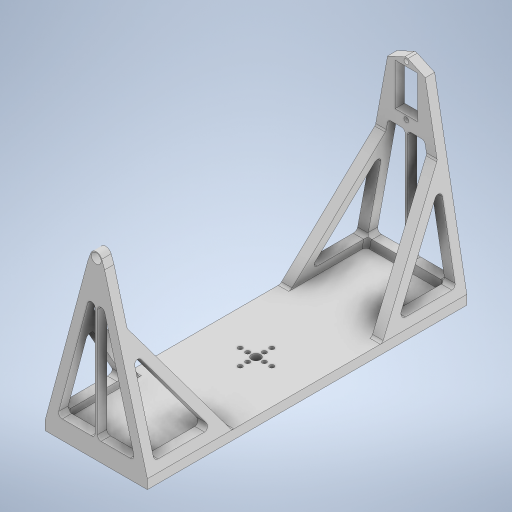
# Autodesk Inventor part: holder
Saved by Autodesk Inventor 2024 (Build 280153000, 153)
## iProperties
Created: 2025-03-10
Part Number: holder
Material: Generic
Document SubType Name: Modeling
Designer: 5454s
Density: 1 g/cm^3
Appearance: Default
Author: 5454s
Autodesk Inventor part; units mm, degrees
ref_plane "YZ Plane" through (0, 0, 0) normal (1, 0, 0) x (0, 1, 0)
ref_plane "XZ Plane" through (0, 0, 0) normal (0, 1, 0) x (-1, 0, 0)
ref_plane "XY Plane" through (0, 0, 0) normal (0, 0, 1) x (1, 0, 0)
sketch "Sketch1" plane through (0, 0, 0) normal (0, 0, 1) x (1, 0, 0)
  line L0 (0, 0) -> (8.8545, 0)
  line L1 (8.8545, 0) -> (8.8545, 85)
  line L2 (8.8545, 85) -> (0, 85)
  line L3 (0, 85) -> (0, 0)
  line L4 (0, 85) -> (-22.7757, 0)
  line L5 (-22.7757, 0) -> (31.6302, 0)
  line L6 (31.6302, 0) -> (8.8545, 85)
  circle A0 centre (4.4273, 88.1) radius 3.1
  line L7 (4.4273, 0) -> (4.4273, 91.736)
  line L8 (7.5273, 88.1) -> (1.3273, 88.1)
  circle A1 centre (4.4273, 88.1) radius 2.6
  line L9 (4.4273, 88.1) -> (1.5142, 89.1603)
  line L10 (1.5142, 89.1603) -> (0, 85)
  line L11 (4.4273, 88.1) -> (7.3403, 89.1603)
  line L12 (7.3403, 89.1603) -> (8.8545, 85)
  line L13 (-16.2596, 5) -> (4.4273, 5)
  line L14 (3.8366, 80) -> (-16.2596, 5)
  line L15 (3.8366, 80) -> (4.4273, 80)
  line L16 (4.4273, 80) -> (5.0179, 80)
  line L17 (5.0179, 80) -> (25.1141, 5)
  line L18 (25.1141, 5) -> (4.4273, 5)
  line L19 (3.8366, 80) -> (3.8366, 5)
  line L20 (5.0179, 80) -> (5.0179, 5)
  point P0 (0, 42.5)
  point P1 (-15.2073, 5)
  point P2 (20.2424, 42.5)
  dimension "d0" = 85
  dimension "d1" = 75
  dimension "d2" = 75
  dimension "d4" = 6.2
  dimension "d6" = 5.2
  dimension "d7" = 20
  dimension "d8" = 70
  dimension "d9" = 20
  dimension "d10" = 70
  dimension "d15" = 54.4059
  dimension "d22" = 5
  dimension "d27" = 5
  dimension "d28" = 5
  constraints: 42 end point, 6 horizontal, 6 point on line, 4 midpoint, 4 perpendicular, 4 point on circle, 2 centre point, 2 parallel, 1 coincident, 1 collinear, 1 tangent, 1 vertical, 1 other
  measures "d0" distance of L0.end L1.end
  measures "d1" angle of L5 L6
  measures "d2" angle of L5 L4
  measures "d4" diameter of A0
  measures "d6" diameter of A1
  measures "d7" angle of L8 L9
  measures "d8" angle of L2 L10
  measures "d9" angle of L8 L11
  measures "d10" angle of L2 L12
  measures "d15" distance of L5.end L4.end
  measures "d22" distance between parallel lines of L5 L13
  measures "d27" distance between parallel lines of L4 L14
  measures "d28" distance between parallel lines of L2 L15
extrude "Extrusion1" add sketch "Sketch1" along normal blind 5 contours L3 L13 L7 L0 | L5 L4 L3 L14 L13 | L7 L18 L1 L0 | L1 L18 L17 L6 L5 | L13 L19 L15 L7 | L7 L16 L20 L18 | L3 L2 L7 L15 L14 | L10 A0 L2 | L7 L2 L1 L17 L16 | A0 L12 L2 | L7 A1 L8 A0 | A0 L8 A1 L7 | L9 A1 L8 A0 | A0 L7 A1 L9 | L8 A1 L11 A0 | A0 L11 A1 L7
fillet "Fillet1" radius 2 6 edges at (5.0179, 5, 2.5) (-16.2596, 5, 2.5) (3.8366, 5, 2.5) (25.1141, 5, 2.5) (3.8366, 80, 2.5) (5.0179, 80, 2.5)
sketch "Sketch2" plane through (-22.7757, 0, 0) normal (0, -1, 0) x (1, 0, 0)
  line L0 (0, 0) -> (54.4059, 0) projected
  line L1 (54.4059, 0) -> (54.4059, 5) projected
  line L2 (0, 5) -> (54.4059, 5) projected
  line L3 (0, 0) -> (0, 5) projected
  line L4 (0, 0) -> (54.4059, 0)
  line L5 (54.4059, 0) -> (54.4059, -144.177)
  line L6 (54.4059, -144.177) -> (0, -144.177)
  line L7 (0, -144.177) -> (0, 0)
  line L8 (54.4059, 0) -> (54.4059, 5) projected
  line L9 (54.4059, -144.177) -> (0, -144.177)
  line L10 (0, -144.177) -> (0, -165.177)
  line L11 (0, -165.177) -> (54.4059, -165.177)
  line L12 (54.4059, -165.177) -> (54.4059, -144.177)
  point P0 (22.7757, 0)
  dimension "d32" = 144.177
  dimension "d34" = 21
  constraints: 16 end point, 4 parallel, 2 collinear, 2 horizontal, 2 perpendicular
  measures "d32" distance of L4.end L5.end
  measures "d34" distance of L9.end L10.end
extrude "Extrusion2" add sketch "Sketch2" along normal blind 5
sketch "Sketch5" plane through (-22.7757, 0, 0) normal (0, 1, 0) x (1, 0, 0)
  line L0 (0, 0) -> (54.4059, 0) projected
  line L1 (54.4059, 165.177) -> (54.4059, 0) projected
  line L2 (0, 165.177) -> (54.4059, 165.177) projected
  line L3 (0, 0) -> (0, 165.177) projected
  line L4 (54.4059, 165.177) -> (0, 165.177)
  line L5 (0, 165.177) -> (0, 160.177)
  line L6 (0, 160.177) -> (54.4059, 160.177)
  line L7 (54.4059, 160.177) -> (54.4059, 165.177)
  point P0 (22.7757, 0)
  dimension "d37" = 5
  constraints: 8 end point, 2 parallel, 1 horizontal, 1 perpendicular, 1 point on line
  measures "d37" distance between parallel lines of L2 L6
extrude "Extrusion3" add sketch "Sketch5" along normal up to surface (91.2 mm away) contours L3 L2 L1 L6
sketch "Sketch9" plane through (31.6302, -5, -165.177) normal (0, 0, -1) x (-1, 0, 0)
  line L0 (31.6302, 90) -> (54.4059, 5) projected
  line L1 (0, 5) -> (22.7757, 90) projected
  circle A0 centre (27.2029, 93.1) radius 2.6 projected
  line L2 (30.116, 94.1603) -> (31.6302, 90) projected
  line L3 (22.7757, 90) -> (24.2899, 94.1603) projected
  arc A1 (30.116, 94.1603) -> (24.2899, 94.1603) centre (27.2029, 93.1) ccw projected
  circle A2 centre (27.2029, 101.3) radius 1.25
  circle A3 centre (27.2029, 74.5) radius 1.25
  line L4 (21.2029, 76.6) -> (33.2029, 76.6)
  line L5 (33.2029, 76.6) -> (33.2029, 99)
  line L6 (33.2029, 99) -> (21.2029, 99)
  line L7 (21.2029, 99) -> (21.2029, 76.6)
  line L8 (0, 5) -> (17.1194, 98.9034)
  circle A4 centre (27.2029, 101.3) radius 2
  line L9 (0, 5) -> (54.4059, 5) projected
  line L10 (25.2029, 101.3) -> (29.2029, 101.3)
  line L11 (27.2029, 101.3) -> (26.3577, 103.1126)
  line L12 (26.3577, 103.1126) -> (17.1194, 98.9034)
  line L13 (27.2029, 101.3) -> (28.0482, 103.1126)
  line L14 (54.4059, 5) -> (37.2029, 98.8882)
  line L15 (28.0482, 103.1126) -> (37.2029, 98.8882)
  point P0 (31.6302, 5)
  point P1 (27.2029, 99)
  point P2 (21.2029, 84.1305)
  point P3 (33.2029, 84.1305)
  dimension "d54" = 8.2
  dimension "d55" = 18.6
  dimension "d56" = 12
  dimension "d57" = 22.4
  dimension "d58" = 2.5
  dimension "d59" = 2.3
  dimension "d60" = 4
  dimension "d62" = 4
  dimension "d63" = 79.668
  dimension "d64" = 65
  dimension "d65" = 65
  dimension "d66" = 124.827
  dimension "d67" = 4
  constraints: 22 end point, 4 point on circle, 3 centre point, 3 vertical alignment, 2 horizontal, 2 parallel, 1 coincident, 1 equal length, 1 equal radius, 1 midpoint, 1 perpendicular
  measures "d54" distance of A0.centre A2.centre
  measures "d55" distance of A3.centre A0.centre
  measures "d56" distance of L4.start L4.end
  measures "d57" distance of L4.end L5.end
  measures "d58" diameter of A2
  measures "d59" distance from line of A2.centre L6
  measures "d60" distance from line of L8 L6.end
  measures "d62" diameter of A4
  measures "d63" angle of L9 L8
  measures "d64" angle of L10 L11
  measures "d65" angle of L10 L13
  measures "d66" angle of L8 L12
  measures "d67" horizontal distance of L14.end L5.end
extrude "Extrusion6" add sketch "Sketch9" against normal up to surface (5 mm away) contours L5 L6 L7 L1 L8 L12 A4 L15 L14 L0 | L13 A2 L11 A4 | A4 L10 A2 L13 | L11 A2 L10 A4 | A4 L10 A2
sketch "Sketch10" plane through (31.6302, -5, -165.177) normal (0, 0, -1) x (-1, 0, 0)
  line L0 (16.6265, 96.2) -> (0, 96.2) projected
  line L1 (0, 96.2) -> (0, 0) projected
  line L2 (54.4059, 0) -> (0, 0) projected
  line L3 (54.4059, 96.2) -> (54.4059, 0) projected
  line L4 (54.4059, 96.2) -> (37.6955, 96.2) projected
  line L5 (37.6955, 96.2) -> (37.2029, 98.8882) projected
  line L6 (37.2029, 98.8882) -> (28.0482, 103.1126) projected
  arc A0 (28.0482, 103.1126) -> (26.3577, 103.1126) centre (27.2029, 101.3) ccw projected
  line L7 (26.3577, 103.1126) -> (17.1194, 98.9034) projected
  line L8 (17.1194, 98.9034) -> (16.6265, 96.2) projected
  circle A1 centre (27.2029, 101.3) radius 1.25 projected
  line L9 (21.2029, 96.2) -> (21.2029, 99) projected
  line L10 (21.2029, 99) -> (33.2029, 99) projected
  line L11 (33.2029, 99) -> (33.2029, 96.2) projected
  line L12 (33.2029, 96.2) -> (21.2029, 96.2) projected
  line L13 (21.2029, 99) -> (33.2029, 99)
  line L14 (33.2029, 99) -> (33.2029, 76.6)
  line L15 (33.2029, 76.6) -> (21.2029, 76.6)
  line L16 (21.2029, 76.6) -> (21.2029, 99)
  circle A2 centre (27.2029, 74.5) radius 1.25
  circle A3 centre (27.2029, 101.3) radius 1.25 projected
  line L17 (31.6302, 90) -> (54.4059, 5) projected
  line L18 (0, 5) -> (22.7757, 90) projected
  line L19 (0, 5) -> (54.4059, 5) projected
  line L20 (17.1194, 98.9034) -> (0, 5)
  line L21 (37.2029, 98.8882) -> (54.4059, 5)
  point P0 (31.6302, 5)
  point P1 (37.6955, 96.2)
  point P2 (21.2029, 96.2)
  dimension "d70" = 22.4
  dimension "d71" = 26.8
  constraints: 12 end point, 2 parallel, 1 centre point, 1 equal radius, 1 horizontal, 1 perpendicular, 1 vertical alignment
  measures "d70" distance of L10.end L14.end
  measures "d71" distance of A2.centre A0.centre
extrude "Extrusion7" cut sketch "Sketch10" against normal blind 10 contours L20 L1 L0 | L16 L12 L14 L15 | L21 L4 L3 | A2
sketch "Sketch11" plane through (31.6302, -5, -165.177) normal (0, 0, -1) x (-1, 0, 0)
  line L0 (47.2152, 12.5176) -> (31.7254, 70.3261) projected
  line L1 (22.6805, 70.3261) -> (7.1907, 12.5176) projected
  arc A0 (26.6123, 69.8085) -> (22.6805, 70.3261) centre (24.6123, 69.8085) ccw projected
  arc A1 (31.7254, 70.3261) -> (27.7936, 69.8085) centre (29.7936, 69.8085) ccw projected
  line L2 (9.1226, 10) -> (24.6123, 10) projected
  line L3 (29.7936, 10) -> (45.2833, 10) projected
  arc A2 (7.1907, 12.5176) -> (9.1226, 10) centre (9.1226, 12) ccw projected
  arc A3 (24.6123, 10) -> (26.6123, 12) centre (24.6123, 12) ccw projected
  arc A4 (27.7936, 12) -> (29.7936, 10) centre (29.7936, 12) ccw projected
  arc A5 (45.2833, 10) -> (47.2152, 12.5176) centre (45.2833, 12) ccw projected
  line L4 (26.6123, 12) -> (26.6123, 69.8085) projected
  line L5 (27.7936, 69.8085) -> (27.7936, 12) projected
  line L6 (6.5161, 10) -> (47.8898, 10)
  circle A6 centre (27.2029, 101.3) radius 1.25 projected
  circle A7 centre (27.2029, 74.5) radius 1.25 projected
  line L7 (17.1194, 98.9034) -> (0, 5) projected
  line L8 (0, 5) -> (0, 0) projected
  line L9 (54.4059, 0) -> (0, 0) projected
  line L10 (54.4059, 5) -> (54.4059, 0) projected
  line L11 (54.4059, 5) -> (37.2029, 98.8882) projected
  line L12 (37.2029, 98.8882) -> (28.0482, 103.1126) projected
  arc A8 (28.0482, 103.1126) -> (26.3577, 103.1126) centre (27.2029, 101.3) ccw projected
  line L13 (26.3577, 103.1126) -> (17.1194, 98.9034) projected
  line L14 (21.2029, 76.6) -> (21.2029, 99) projected
  line L15 (21.2029, 99) -> (33.2029, 99) projected
  line L16 (33.2029, 99) -> (33.2029, 76.6) projected
  line L17 (33.2029, 76.6) -> (21.2029, 76.6) projected
  line L18 (22.6805, 70.3261) -> (22.5418, 69.8085)
  line L19 (22.5418, 69.8085) -> (36.9312, 69.8085)
  line L20 (22.5418, 69.8085) -> (17.4197, 69.8085)
  line L21 (36.9312, 69.8085) -> (29.7936, 69.8085)
  line L22 (6.5161, 10) -> (17.4197, 69.8085)
  line L23 (17.1194, 98.9034) -> (0, 5) projected
  line L24 (54.4059, 0) -> (0, 0) projected
  line L25 (47.8898, 10) -> (36.9312, 69.8085)
  line L26 (54.4059, 5) -> (37.2029, 98.8882) projected
  point P0 (31.6302, 5)
  point P1 (27.7936, 69.8085)
  point P2 (45.2833, 10)
  point P3 (26.6123, 69.8085)
  point P4 (9.1226, 10)
  dimension "d74" = 41.3736
  constraints: 16 end point, 3 parallel, 3 point on line, 2 horizontal, 1 coincident, 1 tangent
  measures "d74" distance of L6.start L6.end
extrude "Extrusion8" cut sketch "Sketch11" against normal blind 10 contours A5 L3 A4 L5 L19 L0 | L0 L19 L25 L6 A5 | L2 A2 L1 L19 L4 A3 | L6 L22 L20 L1 A2
fillet "Fillet2" radius 2 6 edges at (25.1141, 5, -162.677) (-16.2596, 5, -162.677) (14.2105, 64.8085, -162.677) (3.8366, 64.8085, -162.677) (-5.301, 64.8085, -162.677) (5.0179, 64.8085, -162.677)
sketch "Sketch14" plane through (0, 0, 0) normal (0, 0, -1) x (-1, 0, 0)
  line L0 (-1.5142, 89.1603) -> (0, 85) projected
  arc A0 (-1.5142, 89.1603) -> (-7.3403, 89.1603) centre (-4.4273, 88.1) ccw projected
  line L1 (-8.8545, 85) -> (-7.3403, 89.1603) projected
  line L2 (-31.6302, 0) -> (-8.8545, 85) projected
  line L3 (22.7757, 0) -> (-31.6302, 0) projected
  line L4 (0, 85) -> (22.7757, 0) projected
  circle A1 centre (-4.4273, 88.1) radius 2.6 projected
  arc A2 (13.6531, 5) -> (15.585, 7.5176) centre (13.6531, 7) ccw projected
  line L5 (-1.8366, 5) -> (13.6531, 5) projected
  arc A3 (-3.8366, 7) -> (-1.8366, 5) centre (-1.8366, 7) ccw projected
  line L6 (-3.8366, 64.8085) -> (-3.8366, 7) projected
  arc A4 (0.0952, 65.3261) -> (-3.8366, 64.8085) centre (-1.8366, 64.8085) ccw projected
  line L7 (15.585, 7.5176) -> (0.0952, 65.3261) projected
  arc A5 (-7.0179, 5) -> (-5.0179, 7) centre (-7.0179, 7) ccw projected
  line L8 (-22.5076, 5) -> (-7.0179, 5) projected
  arc A6 (-24.4395, 7.5176) -> (-22.5076, 5) centre (-22.5076, 7) ccw projected
  line L9 (-8.9497, 65.3261) -> (-24.4395, 7.5176) projected
  arc A7 (-5.0179, 64.8085) -> (-8.9497, 65.3261) centre (-7.0179, 64.8085) ccw projected
  line L10 (-5.0179, 7) -> (-5.0179, 64.8085) projected
  line L11 (-10.4983, 59.5466) -> (-26.4538, 0)
  line L12 (1.6438, 59.5466) -> (17.5993, 0)
  line L13 (-9.0884, 64.8085) -> (-10.4983, 59.5466)
  line L14 (0.2339, 64.8085) -> (1.6438, 59.5466)
  line L15 (-9.0884, 64.8085) -> (-14.2648, 64.8085)
  line L16 (0.2339, 64.8085) -> (5.4103, 64.8085)
  line L17 (-15.8212, 59) -> (-10.6448, 59)
  line L18 (22.7757, 0) -> (-31.6302, 0) projected
  line L19 (1.7903, 59) -> (6.9667, 59)
  point P0 (0, 0)
  point P1 (-11.6766, 64.8085)
  point P2 (-13.233, 59)
  point P3 (4.3785, 59)
  dimension "d88" = 64.8085
  dimension "d89" = 59
  dimension "d90" = 59
  constraints: 16 end point, 15 point on line, 3 horizontal, 3 midpoint, 2 collinear, 2 parallel
  measures "d88" distance from line of L3 point (-11.677, 64.808)
  measures "d89" distance from line of L18 point (-13.233, 59)
  measures "d90" distance from line of L18 point (4.378, 59)
extrude "Extrusion9" add sketch "Sketch14" along normal blind 40 contours L4 L3 L12 L7 L19 | L17 L9 L11 L3 L2
sketch "Sketch16" plane through (31.6302, -5, 5) normal (1, 0, 0) x (0, 0, -1)
  line L0 (5, 64) -> (5, 90) projected
  line L1 (5, 90) -> (0, 90) projected
  line L2 (0, 5) -> (0, 90) projected
  line L3 (45, 5) -> (0, 5) projected
  line L4 (45, 64) -> (45, 5) projected
  line L5 (5, 69.8085) -> (5, 5)
  line L6 (5, 55.0899) -> (5, 10)
  line L7 (5, 10) -> (35.5694, 10)
  line L8 (35.5694, 10) -> (5, 55.0899)
  line L9 (5, 64) -> (45, 64) projected
  line L10 (5, 64) -> (45, 5)
  dimension "d83" = 5
  dimension "d84" = 0
  dimension "d91" = 5
  constraints: 10 end point, 2 vertical, 1 parallel, 1 perpendicular
  measures "d83" distance between parallel lines of L3 L7
  measures "d84" distance between parallel lines of L5 L6
  measures "d91" distance between parallel lines of L10 L8
extrude "Extrusion10" cut sketch "Sketch16" against normal through all contours L9 L4 L10 | L8 L7 L5
sketch "Sketch17" plane through (-22.7757, 0, -160.177) normal (0, 0, 1) x (1, 0, 0)
  arc A0 (24.6123, 5) -> (26.6123, 7) centre (24.6123, 7) ccw projected
  line L0 (24.6123, 5) -> (8.9159, 5) projected
  arc A1 (6.9486, 7.3605) -> (8.9159, 5) centre (8.9159, 7) ccw projected
  line L1 (6.9486, 7.3605) -> (17.1743, 63.1689) projected
  arc A2 (19.1416, 64.8085) -> (17.1743, 63.1689) centre (19.1416, 62.8085) ccw projected
  line L2 (19.1416, 64.8085) -> (24.6123, 64.8085) projected
  arc A3 (26.6123, 62.8085) -> (24.6123, 64.8085) centre (24.6123, 62.8085) ccw projected
  line L3 (26.6123, 62.8085) -> (26.6123, 7) projected
  line L4 (37.2854, 63.1672) -> (47.4597, 7.3587) projected
  arc A4 (45.4922, 5) -> (47.4597, 7.3587) centre (45.4922, 7) ccw projected
  line L5 (45.4922, 5) -> (29.7936, 5) projected
  arc A5 (27.7936, 7) -> (29.7936, 5) centre (29.7936, 7) ccw projected
  line L6 (27.7936, 7) -> (27.7936, 62.8085) projected
  arc A6 (29.7936, 64.8085) -> (27.7936, 62.8085) centre (29.7936, 62.8085) ccw projected
  line L7 (29.7936, 64.8085) -> (35.3178, 64.8085) projected
  arc A7 (37.2854, 63.1672) -> (35.3178, 64.8085) centre (35.3178, 62.8085) ccw projected
  circle A8 centre (27.2029, 96.3) radius 1.25 projected
  line L8 (33.2029, 94) -> (33.2029, 71.6) projected
  line L9 (33.2029, 71.6) -> (21.2029, 71.6) projected
  line L10 (21.2029, 94) -> (21.2029, 71.6) projected
  line L11 (33.2029, 94) -> (21.2029, 94) projected
  circle A9 centre (27.2029, 69.5) radius 1.25 projected
  line L12 (37.2865, 93.9034) -> (54.4059, 0) projected
  line L13 (28.0482, 98.1126) -> (37.2865, 93.9034) projected
  arc A10 (28.0482, 98.1126) -> (26.3577, 98.1126) centre (27.2029, 96.3) ccw projected
  line L14 (17.2029, 93.8882) -> (26.3577, 98.1126) projected
  line L15 (17.2029, 93.8882) -> (0, 0) projected
  line L16 (54.4059, 0) -> (0, 0) projected
  line L17 (6.5161, 5) -> (47.8898, 5)
  line L18 (6.5161, 5) -> (16.4104, 59)
  line L19 (16.4104, 59) -> (16.4104, 5)
  line L20 (16.4104, 59) -> (10.8105, 59)
  line L21 (16.4104, 59) -> (43.6497, 59)
  line L22 (16.4104, 59) -> (5.6, 0)
  line L23 (37.9954, 59) -> (48.8059, 0)
  line L24 (27.2029, 5) -> (27.2029, 59)
  line L25 (10.8105, 59) -> (43.6497, 59)
  point P0 (22.7757, 0)
  point P1 (6.5161, 5)
  point P2 (17.1743, 63.1689)
  point P3 (47.474, 7.2692)
  point P4 (37.1512, 63.6077)
  point P5 (6.5161, 5)
  point P6 (27.7936, 59)
  point P7 (38.0451, 59)
  dimension "d87" = 54
  constraints: 18 end point, 10 point on line, 3 horizontal, 2 collinear, 2 perpendicular, 1 midpoint, 1 other
  measures "d87" distance of L18.end L19.end
extrude "Extrusion11" add sketch "Sketch17" along normal blind 40 from surface at 0 contours L1 L18 L22 L16 L15 L20 | A4 L4 L21 L12 L16 L23
sketch "Sketch19" plane through (31.6302, -5, 5) normal (1, 0, 0) x (0, 0, -1)
  line L0 (165.177, 64) -> (125.177, 64) projected
  line L1 (125.177, 64) -> (125.177, 5) projected
  line L2 (170.177, 5) -> (125.177, 5) projected
  line L3 (170.177, 98.9034) -> (170.177, 5) projected
  line L4 (170.177, 98.9034) -> (165.177, 98.9034) projected
  line L5 (165.177, 98.9034) -> (165.177, 64) projected
  line L6 (165.177, 64) -> (125.177, 5)
  line L7 (165.177, 64) -> (165.177, 5)
  line L8 (165.177, 55.0899) -> (134.6076, 10)
  line L9 (134.6076, 10) -> (165.177, 10)
  point P0 (5, 5)
  dimension "d99" = 5
  dimension "d100" = 5
  constraints: 8 end point, 3 point on line, 2 perpendicular, 1 parallel
  measures "d99" distance between parallel lines of L6 L8
  measures "d100" distance between parallel lines of L2 L9
extrude "Extrusion13" cut sketch "Sketch19" against normal through all contours L6 L1 L0 | L7 L9 L8
fillet "Fillet4" radius 2 12 edges at (27.7023, 5, -30.5694) (27.9164, 5, -160.177) (-19.0595, 5, -160.177) (-18.8477, 5, -30.5694) (27.7023, 5, 0) (-18.8477, 5, 0) (-19.0595, 5, -129.6076) (27.9164, 5, -129.6076) (15.6205, 50.0899, 0) (-6.766, 50.0899, 0) (19.6961, 50.0899, -160.177) (-10.7978, 50.0899, -160.177)
fillet "Fillet5" radius 2 8 edges at (18.0717, 59, -160.177) (-9.1652, 59, -160.177) (28.8302, 0, -120.177) (-19.9757, 0, -120.177) (29.042, 0, -40) (-20.1875, 0, -40) (13.233, 59, 0) (-4.3785, 59, 0)
fillet "Fillet6" radius 2 4 edges at (-16.6615, 3.5, 0) (-16.5344, 3.5, -160.177) (25.3889, 3.5, -160.177) (25.516, 3.5, 0)
sketch "Sketch20" plane through (-22.7757, -5, 0) normal (0, -1, 0) x (1, 0, 0)
  line L0 (17.2029, -82.5885) -> (37.2029, -82.5885)
  line L1 (37.2029, -82.5885) -> (37.2029, -77.5885)
  line L2 (37.2029, -77.5885) -> (17.2029, -77.5885)
  line L3 (17.2029, -77.5885) -> (17.2029, -82.5885)
  circle A0 centre (22.7529, -80.0885) radius 1.15
  circle A1 centre (31.6529, -80.0885) radius 1.15
  line L4 (17.2029, -80.0885) -> (37.2029, -80.0885)
  circle A2 centre (27.2029, -84.5385) radius 1.15
  circle A3 centre (27.2029, -75.6385) radius 1.15
  circle A4 centre (27.2029, -88.5385) radius 1.15
  circle A5 centre (35.6529, -80.0885) radius 1.15
  circle A6 centre (27.2029, -71.6385) radius 1.15
  circle A7 centre (18.7529, -80.0885) radius 1.15
  line L5 (0, 5) -> (0, -165.177) projected
  line L6 (0, -165.177) -> (54.4059, -165.177) projected
  line L7 (54.4059, -165.177) -> (54.4059, 5) projected
  line L8 (54.4059, 5) -> (0, 5) projected
  line L9 (54.4059, -80.0885) -> (0, -80.0885)
  circle A8 centre (27.2029, -80.0885) radius 2.4
  line L10 (27.2029, -77.5885) -> (27.2029, -71.6385)
  line L11 (27.2029, -71.6385) -> (27.2029, -88.5385)
  line L12 (27.2029, 5) -> (27.2029, -165.177)
  point P0 (22.7757, 0)
  point P1 (27.2029, -80.0885)
  dimension "d108" = 8.9
  dimension "d110" = 4.45
  dimension "d111" = 4.45
  dimension "d112" = 4.45
  dimension "d121" = 8.9
  dimension "d122" = 4.8
  constraints: 18 end point, 10 midpoint, 9 centre point, 3 equal radius, 2 coincident, 2 point on line, 2 vertical alignment, 1 collinear, 1 vertical
  measures "d108" distance of A1.centre A0.centre
  measures "d110" distance of point (27.203, -80.088) A1.centre
  measures "d111" distance of point (27.203, -80.088) A2.centre
  measures "d112" distance of A3.centre point (27.203, -80.088)
  measures "d121" distance of A2.centre A3.centre
  measures "d122" diameter of A8
extrude "Extrusion14" cut sketch "Sketch20" against normal up to surface (5 mm away) contours L11 L4 A8 | A8 L4 L11 | L11 A2 | A2 L11 | A7 L4 | L4 A7 | A8 L11 L4 | L4 L11 A8 | A5 L4 | L4 A5 | L4 A0 | A0 L4 | L4 A1 | A1 L4 | L11 L12 A4 | A4 L12 L11 | L10 A3 | A3 L10 | L12 L10 A6 | A6 L10 L12
body "Solid1"
